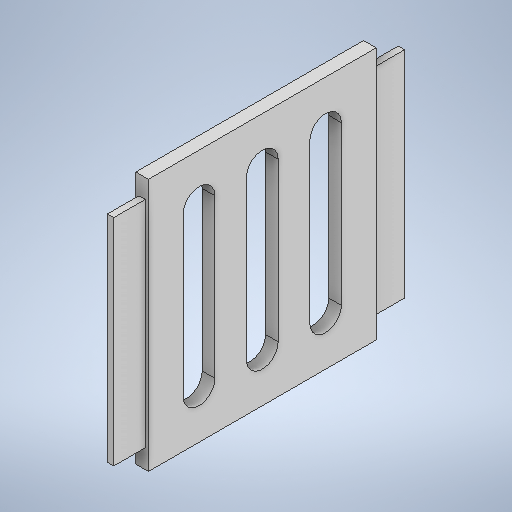
# Autodesk Inventor part: TSU_MM_Wall
Saved by Autodesk Inventor 2025.2 (Build 292293000, 293)
## iProperties
Created: 2025-01-07
Part Number: TSU_MM_Wall
Material: Generic
Document SubType Name: Modeling
Designer: Matt Tidd
Density: 1 g/cm^3
Appearance: Default
Author: Matt Tidd
Autodesk Inventor part; units mm, degrees
ref_plane "YZ Plane" through (0, 0, 0) normal (1, 0, 0) x (0, 1, 0)
ref_plane "XZ Plane" through (0, 0, 0) normal (0, 1, 0) x (-1, 0, 0)
ref_plane "XY Plane" through (0, 0, 0) normal (0, 0, 1) x (1, 0, 0)
sketch "Sketch1" plane through (0, 0, 0) normal (0, 1, 0) x (-1, 0, 0)
  line L0 (0, 0) -> (10, 0)
  line L1 (10, 0) -> (10, -180)
  line L2 (10, -180) -> (0, -180)
  line L3 (0, -180) -> (0, 0)
  dimension "d0" = 10
  dimension "d1" = 180
  constraints: 8 end point, 2 parallel, 1 horizontal, 1 perpendicular
  measures "d0" distance of L1.end L2.end
  measures "d1" distance of L0.end L1.end
extrude "Extrusion1" add sketch "Sketch1" along normal blind 200
sketch "Sketch2" plane through (-10, 0, 0) normal (0, 0, 1) x (1, 0, 0)
  line L0 (10, 0) -> (0, 0) projected
  line L1 (10, 200) -> (0, 200) projected
  line L2 (2.5, 0) -> (7.5, 0)
  line L3 (7.5, 0) -> (7.5, 200)
  line L4 (7.5, 200) -> (2.5, 200)
  line L5 (2.5, 200) -> (2.5, 0)
  line L6 (10, 0) -> (10, 200) projected
  line L7 (0, 200) -> (10, 200)
  line L8 (10, 200) -> (10, 185)
  line L9 (10, 185) -> (0, 185)
  line L10 (0, 185) -> (0, 200)
  line L11 (0, 0) -> (10, 0)
  line L12 (10, 0) -> (10, 15)
  line L13 (10, 15) -> (0, 15)
  line L14 (0, 15) -> (0, 0)
  point P0 (2.5, 15)
  point P1 (7.5, 15)
  point P2 (7.5, 185)
  point P3 (2.5, 185)
  dimension "d4" = 5
  dimension "d5" = 15
  dimension "d6" = 15
  constraints: 24 end point, 6 parallel, 6 point on line, 3 horizontal, 3 perpendicular
  measures "d4" distance of L4.end L3.end
  measures "d5" distance of L7.end L8.end
  measures "d6" distance of L12.end L11.end
extrude "Extrusion2" add sketch "Sketch2" along normal blind 25 contours L13 L5 L9 L3
sketch "Sketch3" plane through (0, 0, -180) normal (0, 0, -1) x (-1, 0, 0)
  line L0 (2.5, 15) -> (7.5, 15)
  line L1 (7.5, 15) -> (7.5, 185)
  line L2 (7.5, 185) -> (2.5, 185)
  line L3 (2.5, 185) -> (2.5, 15)
  point P0 (0, 0)
  dimension "d9" = 5
  dimension "d10" = 170
  constraints: 8 end point, 2 parallel, 1 horizontal, 1 perpendicular
  measures "d9" distance of L2.end L1.end
  measures "d10" distance of L1.end L0.end
extrude "Extrusion3" add sketch "Sketch3" along normal blind 25
sketch "Sketch4" plane through (0, 0, 0) normal (1, 0, 0) x (0, 0, -1)
  line L0 (27.5, 175) -> (52.5, 175)
  line L1 (52.5, 175) -> (52.5, 25)
  line L2 (52.5, 25) -> (27.5, 25)
  line L3 (27.5, 25) -> (27.5, 175)
  line L4 (77.5, 25) -> (102.5, 25)
  line L5 (102.5, 25) -> (102.5, 175)
  line L6 (102.5, 175) -> (77.5, 175)
  line L7 (77.5, 175) -> (77.5, 25)
  line L8 (127.5, 175) -> (152.5, 175)
  line L9 (152.5, 175) -> (152.5, 25)
  line L10 (152.5, 25) -> (127.5, 25)
  line L11 (127.5, 25) -> (127.5, 175)
  point P0 (0, 0)
  dimension "d13" = 25
  dimension "d14" = 150
  dimension "d15" = 25
  dimension "d16" = 25
  constraints: 24 end point, 6 parallel, 4 point on line, 3 horizontal, 3 perpendicular
  measures "d13" distance of L1.end L2.end
  measures "d14" distance of L0.end L1.end
  measures "d15" distance of L6.end L5.end
  measures "d16" distance of L9.end L10.end
extrude "Extrusion4" cut sketch "Sketch4" against normal blind 10
fillet "Fillet1" radius 12.5 12 edges at (-5, 175, -77.5) (-5, 175, -102.5) (-5, 175, -152.5) (-5, 175, -127.5) (-5, 175, -27.5) (-5, 175, -52.5) (-5, 25, -102.5) (-5, 25, -52.5) (-5, 25, -27.5) (-5, 25, -77.5) (-5, 25, -127.5) (-5, 25, -152.5)
body "Solid1"
